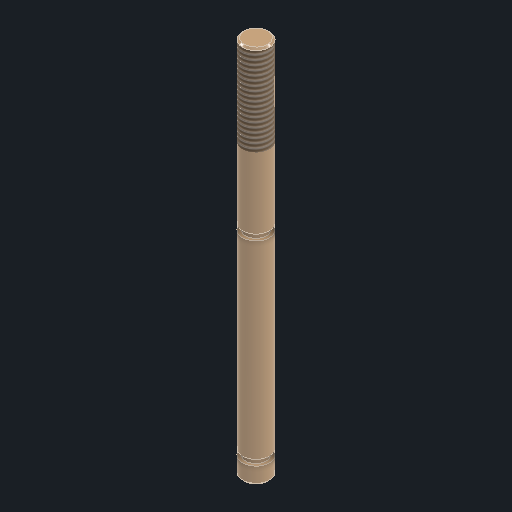
# Autodesk Inventor part: Ball Track Support
Saved by Autodesk Inventor 2027.1 (Build 311270010, 270A)
## iProperties
Created: 2025-09-16
Material: Stainless Steel
Document SubType Name: Modeling
Designer: SD
Density: 8 g/cm^3
Appearance: Brindle
Mass: 2.34186 g
Surface Area: 4.16462 cm^2
Volume: 0.292732 cm^3
Project: Automatic Tea Steeping mechanism
Part Number: Ball Track Support
Length: 42.000 mm
BOM-Mass: 0.00260
BOM-Area: 0.000
Diameter: 3.000 mm
Procurement: Fabricate - 2nd round
Build Stage: 3
Preferred Material: 303 Stainless Steel
Author: SD
Title: Ball Track Support
Autodesk Inventor part; units mm, degrees
ref_plane "YZ Plane" through (0, 0, 0) normal (1, 0, 0) x (0, 1, 0)
ref_plane "XZ Plane" through (0, 0, 0) normal (0, 1, 0) x (-1, 0, 0)
ref_plane "XY Plane" through (0, 0, 0) normal (0, 0, 1) x (1, 0, 0)
sketch "Sketch4" plane through (0, 0, 0) normal (0, 1, 0) x (-1, 0, 0)
  circle A0 centre (0, 0) radius 1.5
  constraints: 1 centre point, 1 coincident, 1 other
extrude "Extrusion2" add sketch "Sketch4" along normal mid plane 42
thread "Thread1" size "M3x0.5" class "6g" standard "ANSI Metric M Profile" length 10
chamfer "Chamfer1" distance 0.2 angle 45 2 edges at (1.5, 21, 0) (1.5, -21, 0)
sketch "Sketch14" plane through (0, 0, 0) normal (1, 0, 0) x (0, 1, 0)
  line L0 (-20.8, -1.5) -> (20.8, -1.5) projected
  line L1 (3.15, -1.5) -> (2.5, -1.5)
  line L2 (2.5, -1.5) -> (2.5, -1.15)
  line L3 (2.5, -1.15) -> (3.15, -1.15)
  line L4 (3.15, -1.15) -> (3.15, -1.5)
  line L5 (-21, -1.3) -> (-21, 1.3) projected
  line L6 (-21, 0) -> (13, 0) construction
  line L7 (-20.8, -1.5) -> (20.8, -1.5) projected
  line L8 (-18.5, -1.5) -> (-19.15, -1.5)
  line L9 (-19.15, -1.5) -> (-19.15, -1.15)
  line L10 (-19.15, -1.15) -> (-18.5, -1.15)
  line L11 (-18.5, -1.15) -> (-18.5, -1.5)
  point P0 (0, 0)
  point P1 (-19.15, -1.5)
  dimension "d105" = 1.15
  dimension "d106" = 0.65
  dimension "d107" = 23.5
  dimension "d109" = 0.65
  dimension "d110" = 1.15
  dimension "d111" = 21
  constraints: 18 end point, 4 parallel, 3 horizontal, 2 perpendicular, 2 point on line, 1 midpoint
  measures "d105" distance between parallel lines of L6 L3
  measures "d106" distance between parallel lines of L2 L4
  measures "d107" distance between parallel lines of L5 L2
  measures "d109" distance between parallel lines of L9 L11
  measures "d110" distance between parallel lines of L6 L10
  measures "d111" distance between parallel lines of L11 L2
revolve "Revolution1" cut sketch "Sketch14" angle 360 about axis through (0, -21, 0) along (0, 1, 0)
equation "\"d109\" = d106"
equation "\"d110\" = d105"
body "Solid2"
